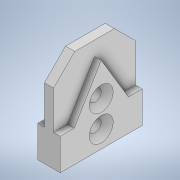
# Autodesk Inventor part: Traingular Hopper Connector
Saved by Autodesk Inventor 2022 (Build 260153000, 153)
## iProperties
Created: 2022-09-14
Part Number: Traingular Hopper Connector
Material: Generic
Document SubType Name: Modeling
Designer: tecssupport
Density: 1 g/cm^3
Appearance: Default
Author: tecssupport
Autodesk Inventor part; units mm, degrees
ref_plane "YZ Plane" through (0, 0, 0) normal (1, 0, 0) x (0, 1, 0)
ref_plane "XZ Plane" through (0, 0, 0) normal (0, 1, 0) x (-1, 0, 0)
ref_plane "XY Plane" through (0, 0, 0) normal (0, 0, 1) x (1, 0, 0)
sketch "Sketch1" plane through (0, 0, 0) normal (1, 0, 0) x (0, 1, 0)
  line L0 (22.5, 15.5) -> (0, 15.5)
  line L1 (0, 15.5) -> (0, -15.5)
  line L2 (0, -15.5) -> (22.5, -15.5)
  line L3 (22.5, -15.5) -> (22.5, 15.5)
  line L4 (0, -21.7) -> (0, 21.7) projected
  point P0 (0, 0)
  point P1 (22.5, 0)
  dimension "d0" = 31
  dimension "d1" = 22.5
  constraints: 8 end point, 2 parallel, 1 collinear, 1 horizontal, 1 horizontal alignment, 1 midpoint, 1 perpendicular
  measures "d0" distance between parallel lines of L2 L0
  measures "d1" distance of L1.end L2.end
extrude "Extrusion1" add sketch "Sketch1" along normal mid plane 3.5
sketch "Sketch2" plane through (1.75, 0, 0) normal (1, 0, 0) x (0, 0, -1)
  line L0 (-10.2455, 0) -> (0, 17.076)
  line L1 (0, 17.076) -> (10.2455, 0)
  line L2 (-15.5, 0) -> (15.5, 0) projected
  point P0 (0, 0)
  dimension "d31" = 20.491
  dimension "d33" = 17.076
  constraints: 4 end point, 2 point on line, 1 equal length, 1 vertical alignment
  measures "d31" distance of L1.end L0.start
  measures "d33" vertical distance of L1.end L0.end
extrude "Extrusion4" add sketch "Sketch2" along normal blind 2.5
mirror "Mirror2" about plane through (0, 0, 0) normal (1, 0, 0) of "Extrusion4"
sketch "Sketch7" plane through (-1.75, 0, -15.5) normal (0, -1, 0) x (1, 0, 0)
  line L0 (0, 0) -> (3.5, 0) projected
  line L1 (3.5, 5.2545) -> (3.5, 0) projected
  line L2 (3.5, 5.2545) -> (6, 5.2545) projected
  line L3 (6, 25.7455) -> (6, 5.2545) projected
  line L4 (3.5, 25.7455) -> (6, 25.7455) projected
  line L5 (3.5, 31) -> (3.5, 25.7455) projected
  line L6 (0, 31) -> (3.5, 31) projected
  line L7 (0, 25.7455) -> (0, 31) projected
  line L8 (0, 25.7455) -> (-2.5, 25.7455) projected
  line L9 (-2.5, 25.7455) -> (-2.5, 5.2545) projected
  line L10 (0, 5.2545) -> (-2.5, 5.2545) projected
  line L11 (0, 0) -> (0, 5.2545) projected
  point P0 (1.75, 15.5)
extrude "Extrusion5" add sketch "Sketch7" along normal blind 12
sketch "Sketch8" plane through (4.25, 0, -10.2455) normal (0, 0, -1) x (-1, 0, 0)
  line L0 (2.5, 0) -> (0, 0) projected
  line L1 (0, 0) -> (0, -12) projected
  line L2 (2.5, -12) -> (0, -12) projected
  line L3 (2.5, 0) -> (2.5, -12) projected
  point P0 (4.25, 0)
extrude "Extrusion6" add sketch "Sketch8" along normal up to surface (5.2545 mm away)
mirror "Mirror3" about plane through (0, 0, 0) normal (0, 0, 1) of "Extrusion6"
mirror "Mirror4" about plane through (0, 0, 0) normal (1, 0, 0) of "Extrusion6", "Mirror3"
sketch "Sketch9" plane through (4.25, 0, 0) normal (1, 0, 0) x (0, 0, -1)
  line L0 (0, 17.076) -> (-10.2455, 0) construction
  line L1 (0, 17.076) -> (0, -12) construction
  line L2 (-15.5, -12) -> (15.5, -12) construction
  line L3 (-5.1228, 8.538) -> (5.1227, 8.538) construction
  line L4 (0, 17.076) -> (10.2455, 0) construction
  line L5 (-7.5227, 4.538) -> (7.5227, 4.538) construction
  line L6 (-13.5227, -5.462) -> (13.5227, -5.462) construction
  point P0 (0, 0)
  dimension "d40" = 4
  dimension "d50" = 10
  constraints: 8 end point, 4 point on line, 3 midpoint, 2 parallel
  measures "d40" distance between parallel lines of L3 L5
  measures "d50" distance between parallel lines of L5 L6
hole "Hole3" at (4.25, 4.538, 0) direction (-1, 0, 0) diameter 4.5 end through all countersink diameter 9 countersink angle 90
hole "Hole4" at (4.25, -5.462, 0) direction (-1, 0, 0) diameter 4.5 end through all countersink diameter 9 countersink angle 90
chamfer "Chamfer1" distance 8 angle 45 2 edges at (0, 22.5, 15.5) (0, 22.5, -15.5)
body "Solid1"
